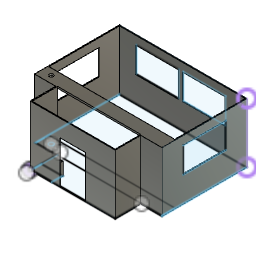
Project (Autodesk Fusion 360 design; units mm, degrees)
Autodesk Fusion 360 part; units mm, degrees
sketch "Schizzo1" plane through (0, 0, 0) normal (0, 0, 1) x (1, 0, 0)
  line L0 (5, 0) -> (115, 0)
  line L1 (120, 5) -> (120, 85)
  line L2 (115, 90) -> (5, 90)
  line L3 (0, 85) -> (0, 5)
  line L4 (12.35, 77.6) -> (83.85, 77.6)
  line L5 (83.85, 77.6) -> (83.85, 67.4089)
  line L6 (83.85, 52.6) -> (12.35, 52.6)
  line L7 (12.35, 52.6) -> (12.35, 77.6)
  line L8 (12.25, 46.5) -> (51.75, 46.5)
  line L9 (51.75, 26.75) -> (51.75, 7)
  line L10 (51.75, 7) -> (12.25, 7)
  line L11 (12.25, 7) -> (12.25, 46.5)
  circle A0 centre (100, 26.75) radius 3.7
  circle A1 centre (100, 67.4089) radius 2.5
  arc A2 (5, 90) -> (0, 85) centre (5, 85) ccw
  arc A3 (120, 85) -> (115, 90) centre (115, 85) ccw
  arc A4 (115, 0) -> (120, 5) centre (115, 5) ccw
  arc A5 (0, 5) -> (5, 0) centre (5, 5) ccw
  line L12 (83.85, 67.4089) -> (83.85, 52.6)
  line L13 (51.75, 46.5) -> (51.75, 26.75)
  line L14 (3, 85) -> (3, 5)
  arc A6 (3, 5) -> (5, 3) centre (5, 5) ccw
  line L15 (5, 3) -> (115, 3)
  arc A7 (115, 3) -> (117, 5.0001) centre (115, 5) ccw
  line L16 (117, 5.0001) -> (117, 85)
  arc A8 (117, 85) -> (115, 87) centre (115, 85) ccw
  line L17 (115, 87) -> (5, 87)
  arc A9 (5, 87) -> (3, 85) centre (5, 85) ccw
  line L18 (2, 85) -> (2, 5)
  arc A10 (2, 5) -> (5, 2) centre (5, 5) ccw
  line L19 (5, 2) -> (115, 2)
  arc A11 (115, 2) -> (118, 5) centre (115, 5) ccw
  line L20 (118, 5) -> (118, 85)
  arc A12 (118, 85) -> (115, 88) centre (115, 85) ccw
  line L21 (115, 88) -> (5, 88)
  arc A13 (5, 88) -> (2, 85) centre (5, 85) ccw
  circle A14 centre (56.5, 44.25) radius 1.65
  circle A15 centre (56.6, 9.45) radius 1.65
  line L22 (8, 83) -> (88, 83)
  line L23 (88, 83) -> (88, 47)
  line L24 (88, 47) -> (8, 47)
  line L25 (8, 47) -> (8, 83)
  circle A16 centre (10.5, 80.5) radius 1.65
  circle A17 centre (85.5, 49.5) radius 1.65
  line L26 (51.75, 7) -> (114.9964, 7) construction
  line L27 (114.9964, 7) -> (114.9964, 19.7951) construction
  line L28 (114.9964, 19.7951) -> (51.75, 19.7951) construction
  line L29 (51.75, 19.7951) -> (51.75, 7) construction
  circle A18 centre (85.5, 49.5) radius 2.15
  circle A19 centre (10.5, 80.5) radius 2.15
  circle A20 centre (56.6, 9.45) radius 2.15
  circle A21 centre (56.5, 44.25) radius 2.15
  point P0 (120, 0)
  point P1 (0, 90)
  dimension "d1" = 90
  dimension "d2" = 120
  dimension "d3" = 71.5
  dimension "d4" = 25
  dimension "d7" = 39.5
  dimension "d8" = 39.5
  dimension "d10" = 7.4
  dimension "d11" = 5
  dimension "d13" = 5
  dimension "d14" = 5
  dimension "d15" = 5
  dimension "d16" = 5
  dimension "d22" = 1
  dimension "d23" = -2
  dimension "d29" = 3.3
  dimension "d31" = 3.3
  dimension "d36" = 44.35
  dimension "d37" = 44.25
  dimension "d38" = 2.25
  dimension "d39" = 2.45
  dimension "d41" = 19.75
  dimension "d44" = 20
  dimension "d45" = 20
  dimension "d46" = 80
  dimension "d47" = 36
  dimension "d48" = 3.3
  dimension "d50" = 3.3
  dimension "d51" = 2.5
  dimension "d53" = 2.5
  dimension "d54" = 5.4
  dimension "d55" = 4.35
  dimension "d56" = 2.5
  dimension "d57" = 2.5
  dimension "d59" = 7
  dimension "d60" = 7
  dimension "d61" = 8
  dimension "d62" = 5
  dimension "d76" = 0.1
  dimension "d77" = 0.5
  dimension "d78" = 0.5
  dimension "d79" = 0.5
  dimension "d80" = 0.5
  text T0 "Salvatore Montagna\n1000080223" font "Arial" height 5 align right middle in box 63.2464 x 12.7951 at (51.75, 7) x (1, 0) y (0, 1) spacing 1 kerned
  constraint horizontal L0
  constraint vertical L1
  constraint horizontal L2
  constraint vertical L3
  constraint horizontal L4
  constraint vertical L5
  constraint horizontal L6
  constraint vertical L7
  constraint vertical L9
  constraint horizontal L10
  constraint vertical L11
  constraint horizontal A0.centre L9.start
  constraint horizontal A1.centre L5.end
  constraint coincident P1 L2
  constraint coincident P1 L3
  constraint tangent L2 A2
  constraint tangent L3 A2
  constraint tangent L1 A3
  constraint tangent L2 A3
  constraint coincident P0 L0
  constraint coincident P0 L1
  constraint tangent L0 A4
  constraint tangent L1 A4
  constraint coincident origin L0
  constraint coincident origin L3
  constraint tangent L0 A5
  constraint tangent L3 A5
  constraint vertical L12
  constraint vertical L13
  constraint horizontal L22
  constraint vertical L23
  constraint horizontal L24
  constraint vertical L25
  constraint coincident L9.end
  constraint coincident L9
  measures "d1" distance of origin P1
  measures "d2" distance of origin P0
  measures "d3" distance of L6.start L6.end
  measures "d4" distance of L4.end L6.start
  measures "d7" distance of L8.start L10.end
  measures "d8" distance of L9.end L10.end
  measures "d10" diameter of A0
  measures "d11" diameter of A1
  measures "d13" radius of A2
  measures "d14" radius of A3
  measures "d15" radius of A4
  measures "d16" radius of A5
  measures "d22" distance of L15 L19
  measures "d29" diameter of A14
  measures "d31" diameter of A15
  measures "d36" distance of L11 A15.centre
  measures "d37" distance of L11 A14.centre
  measures "d38" distance of L8 A14.centre
  measures "d39" vertical distance of L9.end A15.centre
  measures "d41" distance of L10 A0.centre
  measures "d44" distance of L1 A0.centre
  measures "d45" distance of L1 A1.centre
  measures "d46" distance of L23 L25
  measures "d47" distance of L22.end L23.end
  measures "d48" diameter of A16
  measures "d50" diameter of A17
  measures "d51" distance of L22 A16.centre
  measures "d53" distance of L24 A17.centre
  measures "d54" distance of L4 L22
  measures "d55" distance of L7 L25
  measures "d56" distance of L25 A16.centre
  measures "d57" distance of L23 A17.centre
  measures "d59" distance of L0 L10
  measures "d60" distance of L2 L22
  measures "d61" distance of L3 L25
  measures "d76" distance of L7 L11
extrude "Estrusione4" add sketch "Schizzo1" against normal blind 1.5 contours L0 L1 L2 L3 A2 A3 A4 A5 | L14 A6 L15 A7 L16 A8 L17 A9 | L18 A10 L19 A11 L20 A12 L21 A13 | L22 L23 L24 L25 | A18 | A19 | A20 | A21 makes body 1
extrude "Estrusione6" cut sketch "Schizzo1" along normal blind 0.5 text T0 bodies 1
extrude "Estrusione7" cut sketch "Schizzo1" against normal blind 1 text T0 bodies 1
extrude "Estrusione8" add sketch "Schizzo1" against normal blind 6 contours L18 A10 L19 A11 L20 A12 L21 A13 bodies 1
extrude "Estrusione11" add sketch "Schizzo1" against normal blind 6.5 contours A18 | A19 bodies 1
extrude "Estrusione12" add sketch "Schizzo1" against normal blind 4.5 contours A20 | A21 bodies 1
sketch "Schizzo2" plane through (0, 0, 0) normal (0, 0, 1) x (1, 0, 0)
  line L0 (120, 5) -> (120, 85)
  line L1 (2, 85) -> (2, 5)
  line L2 (5, 2) -> (115, 2)
  line L3 (118, 5) -> (118, 85)
  arc A0 (115, 2) -> (118, 5) centre (115, 5) ccw
  line L4 (5, 0) -> (115, 0)
  line L5 (115, 90) -> (5, 90)
  arc A1 (0, 5) -> (5, 0) centre (5, 5) ccw
  line L6 (0, 85) -> (0, 5)
  arc A2 (5, 90) -> (0, 85) centre (5, 85) ccw
  arc A3 (2, 5) -> (5, 2) centre (5, 5) ccw
  arc A4 (5, 88) -> (2, 85) centre (5, 85) ccw
  arc A5 (115, 0) -> (120, 5) centre (115, 5) ccw
  arc A6 (118, 85) -> (115, 88) centre (115, 85) ccw
  arc A7 (120, 85) -> (115, 90) centre (115, 85) ccw
  line L7 (115, 88) -> (5, 88)
  point P0 (120, 0)
  point P1 (0, 90)
  dimension "d90" = -2
  dimension "d95" = 90
  dimension "d96" = 120
  dimension "d103" = 5
  dimension "d104" = 5
  dimension "d105" = 5
  dimension "d106" = 5
  constraint horizontal L4
  constraint vertical L0
  constraint horizontal L5
  constraint vertical L6
  constraint coincident P1 L5
  constraint coincident P1 L6
  constraint tangent L5 A2
  constraint tangent L6 A2
  constraint tangent L0 A7
  constraint tangent L5 A7
  constraint coincident P0 L4
  constraint coincident P0 L0
  constraint tangent L4 A5
  constraint tangent L0 A5
  constraint coincident origin L4
  constraint coincident origin L6
  constraint tangent L4 A1
  constraint tangent A1 L6
  measures "d95" distance of P1 origin
  measures "d96" distance of P0 origin
  measures "d103" radius of A2
  measures "d104" radius of A7
  measures "d105" radius of A5
  measures "d106" radius of A1
extrude "Estrusione13" add sketch "Schizzo2" along normal blind 2 separate body contours L1 L2 L3 A0 A3 A4 A6 L7 makes body 2
extrude "Estrusione14" add sketch "Schizzo2" along normal blind 50.5 bodies 2
sketch "Schizzo3" plane through (0, 0, 0) normal (-1, 0, 0) x (0, -1, 0)
  line L0 (-85, 0) -> (-5, 0)
  line L1 (-5, 0) -> (-5, 50.5)
  line L2 (-5, 50.5) -> (-85, 50.5)
  line L3 (-85, 50.5) -> (-85, 0)
  line L4 (-12, 5) -> (-38, 5)
  line L5 (-40, 7) -> (-40, 23)
  line L6 (-38, 25) -> (-12, 25)
  line L7 (-10, 23) -> (-10, 7)
  arc A0 (-38, 25) -> (-40, 23) centre (-38, 23) ccw
  arc A1 (-10, 23) -> (-12, 25) centre (-12, 23) ccw
  arc A2 (-40, 7) -> (-38, 5) centre (-38, 7) ccw
  arc A3 (-12, 5) -> (-10, 7) centre (-12, 7) ccw
  dimension "d135" = 2
  dimension "d136" = 2
  dimension "d137" = 2
  dimension "d138" = 2
  constraint horizontal L4
  constraint vertical L5
  constraint horizontal L6
  constraint vertical L7
  constraint tangent L5 A0
  constraint tangent L6 A0
  constraint tangent L6 A1
  constraint tangent L7 A1
  constraint tangent L4 A2
  constraint tangent L5 A2
  constraint tangent L4 A3
  constraint tangent L7 A3
  measures "d135" radius of A0
  measures "d136" radius of A1
  measures "d137" radius of A2
  measures "d138" radius of A3
extrude "Estrusione15" cut sketch "Schizzo3" against normal blind 2 contours L4 L5 L6 L7 A0 A1 A2 A3 bodies 2
sketch "Schizzo4" plane through (0, 0, 0) normal (0, 0, 1) x (1, 0, 0)
  line L0 (0, 0) -> (100, 0)
  line L1 (100, 0) -> (100, 30)
  line L2 (0, 30) -> (0, 0)
  line L3 (0, 35) -> (0, 30)
  line L4 (125, 30) -> (125, 130)
  line L5 (125, 130) -> (-25, 130)
  line L6 (-25, 130) -> (-25, 30)
  line L7 (124, 129) -> (-24, 129)
  line L8 (-24, 129) -> (-24, 31)
  line L9 (124, 31) -> (124, 129)
  line L10 (-24, 31) -> (1.2329, 31)
  line L11 (100, 31) -> (124, 31)
  line L12 (1.233, 1) -> (99, 1)
  line L13 (99, 1) -> (99, 31)
  arc A0 (1.233, 31) -> (1.2329, 31) centre (1.2329, -5.4434) ccw
  line L14 (100, 30) -> (125, 30)
  line L15 (-25, 30) -> (0, 30)
  line L16 (124, 31) -> (124, 46)
  line L17 (124, 46) -> (-24, 46)
  line L18 (-24, 46) -> (-24, 31)
  line L19 (1.233, 31) -> (1.233, 1)
  line L20 (-24, 31) -> (1.2329, 31)
  line L21 (99, 31) -> (124, 31)
  line L22 (1.2329, 31) -> (1.233, 31)
  line L23 (1.233, 31) -> (99, 31)
  circle A1 centre (-13.7208, 38.5) radius 2.5
  line L24 (1.233, 1) -> (24.733, 1)
  line L25 (24.733, 1) -> (24.733, 12)
  line L26 (24.733, 12) -> (1.233, 12)
  line L27 (1.233, 12) -> (1.233, 1)
  line L28 (0.233, 0) -> (25.733, 0)
  line L29 (25.733, 0) -> (25.733, 13)
  line L30 (25.733, 13) -> (0.233, 13)
  line L31 (0.233, 13) -> (0.233, 0)
  dimension "d141" = 100
  dimension "d143" = 100
  dimension "d145" = 150
  dimension "d149" = 15
  dimension "d152" = 30
  dimension "d168" = 5
  dimension "d171" = 23.5
  dimension "d172" = 11
  dimension "d173" = 1
  dimension "d177" = 7.5
  constraint horizontal L0
  constraint vertical L1
  constraint vertical L2
  constraint coincident L0.start L2.end
  constraint vertical L3
  constraint horizontal L15
  constraint vertical L4
  constraint horizontal L5
  constraint vertical L6
  constraint tangent L10 A0
  constraint collinear L14 L15
  constraint horizontal L20
  constraint vertical L16
  constraint horizontal L17
  constraint vertical L18
  constraint coincident L9 L16.end
  constraint collinear L11 L20
  constraint horizontal L10.end A0.start
  constraint coincident L13.end L20
  constraint perpendicular L12 L19
  constraint horizontal L24
  constraint vertical L25
  constraint horizontal L26
  constraint vertical L27
  constraint perpendicular L13 L21
  measures "d141" distance of L0.start L0.end
  measures "d143" distance of L6.end L5.end
  measures "d145" distance of L4 L6
  measures "d149" distance of L8.end L17.end
  measures "d152" distance of L0.end L1.end
  measures "d168" diameter of A1
  measures "d171" distance of L25.end L26.end
  measures "d172" distance of L24.end L25.end
  measures "d177" distance of L10 A1.centre
extrude "Estrusione16" add sketch "Schizzo4" along normal blind 70 separate body contours L0 L2 L3 A0 L19 L30 L31 | L0 L12 L19 L24 L27 L28 L29 L30 L31 | L3 A0 L15 | L0 L12 A0 L29 | L0 L1 L3 L4 L5 L6 L7 L8 L9 L10 L11 L12 L13 A0 L14 L15 L16 L18 L20 L21 | L3 L10 A0 L20 makes body 3
sketch "Schizzo5" plane through (0, 0, 0) normal (0, -1, 0) x (1, 0, 0)
  line L0 (0, 0) -> (100, 0)
  line L1 (100, 0) -> (100, 70)
  line L2 (100, 70) -> (0, 70)
  line L3 (0, 70) -> (0, 0)
  line L4 (35, 0) -> (65, 0)
  line L5 (65, 0) -> (65, 50)
  line L6 (65, 50) -> (35, 50)
  line L7 (35, 50) -> (35, 0)
  constraint horizontal L4
  constraint vertical L5
  constraint horizontal L6
  constraint vertical L7
  constraint coincident L0 L4.start
extrude "Estrusione17" add sketch "Schizzo4" along normal blind 2 from surface at 68 contours L8 L9 L10 L11 L16 L17 L18 L20 L21 L23 | A1 bodies 3
extrude "Estrusione18" cut sketch "Schizzo5" against normal blind 1 contours L0 L4 L5 L6 L7 bodies 3
sketch "Schizzo6" plane through (0, 130, 0) normal (0, 1, 0) x (-1, 0, 0)
  line L0 (-125, 0) -> (25, 0)
  line L1 (25, 0) -> (25, 70)
  line L2 (25, 70) -> (-125, 70)
  line L3 (-125, 70) -> (-125, 0)
  line L4 (-100, 60) -> (-50, 60)
  line L5 (-50, 60) -> (-50, 30)
  line L6 (-50, 30) -> (-100, 30)
  line L7 (-100, 30) -> (-100, 60)
  line L8 (-45, 30) -> (5, 30)
  line L9 (5, 30) -> (5, 60)
  line L10 (5, 60) -> (-45, 60)
  line L11 (-45, 60) -> (-45, 30)
  dimension "d158" = 50
  dimension "d159" = 30
  dimension "d160" = 30
  dimension "d161" = 30
  constraint horizontal L4
  constraint vertical L5
  constraint horizontal L6
  constraint vertical L7
  constraint horizontal L8
  constraint vertical L9
  constraint horizontal L10
  constraint vertical L11
  measures "d158" distance of L5.end L6.end
  measures "d159" distance of L4.start L6.end
  measures "d160" distance of L8.end L9.end
  measures "d161" distance of L0 L8
sketch "Schizzo7" plane through (125, 0, 0) normal (1, 0, 0) x (0, 1, 0)
  line L0 (30, 0) -> (130, 0)
  line L1 (130, 0) -> (130, 70)
  line L2 (130, 70) -> (30, 70)
  line L3 (30, 70) -> (30, 0)
  line L4 (55, 60) -> (105, 60)
  line L5 (105, 60) -> (105, 30)
  line L6 (105, 30) -> (55, 30)
  line L7 (55, 30) -> (55, 60)
  line L8 (130, 70) -> (130, 0)
  dimension "d162" = 50
  dimension "d163" = 30
  dimension "d176" = 75
  constraint horizontal L4
  constraint vertical L5
  constraint horizontal L6
  constraint vertical L7
  measures "d162" distance of L5.end L6.end
  measures "d163" distance of L4.end L5.end
  measures "d176" distance of L7 L8
extrude "Estrusione19" cut sketch "Schizzo6" against normal blind 1 contours L4 L5 L6 L7 | L8 L9 L10 L11 bodies 3
extrude "Estrusione20" cut sketch "Schizzo7" against normal blind 150 contours L4 L5 L6 L7 bodies 3
extrude "Estrusione21" cut sketch "Schizzo4" along normal blind 70 contours A1 bodies 3
extrude "Estrusione22" add sketch "Schizzo4" along normal blind 15 contours L12 L19 L25 L26 L29 L30 bodies 3
hidden bodies 1 2
equation "d41 = ( 39.50 / 2 ) * 1 mm"
equation "d74 = -4.50 mm - 1.5 mm"
equation "d85 = -1.5 mm - 5 mm"
equation "d87 = -1.5 mm - 3 mm"
named bodies: "Tappo", "Custodia", "Casa"
